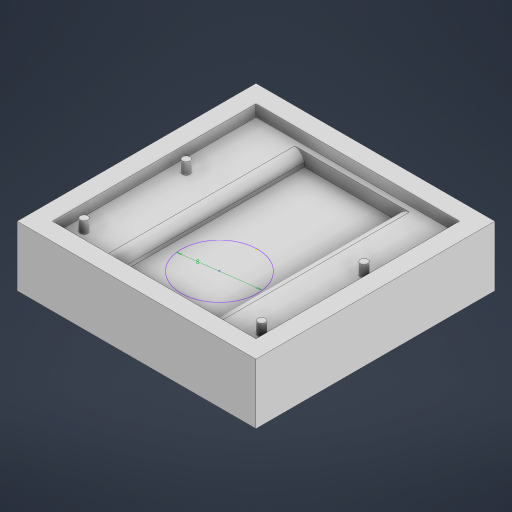
# Autodesk Inventor part: Camera
Saved by Autodesk Inventor 2023.2 (Build 272271030, 271C)
## iProperties
Created: 2025-01-26
Part Number: Camera
Material: Типовые
Document SubType Name: Modeling
Designer: Коноваленко
Density: 1 g/cm^3
Appearance: По умолчанию
Author: Коноваленко
Autodesk Inventor part; units mm, degrees
ref_plane "YZ Plane" through (0, 0, 0) normal (1, 0, 0) x (0, 1, 0)
ref_plane "XZ Plane" through (0, 0, 0) normal (0, 1, 0) x (-1, 0, 0)
ref_plane "XY Plane" through (0, 0, 0) normal (0, 0, 1) x (1, 0, 0)
sketch "Эскиз1" plane through (0, 0, 0) normal (0, 1, 0) x (-1, 0, 0)
  line L0 (12.5, 12.5) -> (-12.5, 12.5)
  line L1 (-12.5, 12.5) -> (-12.5, -12.5)
  line L2 (-12.5, -12.5) -> (12.5, -12.5)
  line L3 (12.5, -12.5) -> (12.5, 12.5)
  line L4 (12.5, 12.5) -> (-12.5, -12.5) construction
  point P0 (0, 0)
  point P1 (0, 0)
  dimension "d0" = 25
  dimension "d1" = 25
  constraints: 10 end point, 2 parallel, 1 coincident, 1 horizontal, 1 midpoint, 1 perpendicular
  measures "d0" distance of L2.end L1.end
  measures "d1" distance of L1.end L0.end
extrude "Выдавливание1" add sketch "Эскиз1" along normal blind 6.3
sketch "Эскиз2" plane through (0, 6.3, 0) normal (0, 1, 0) x (1, 0, 0)
  line L0 (-10.65, -10.65) -> (10.65, -10.65)
  line L1 (10.65, -10.65) -> (10.65, 10.65)
  line L2 (10.65, 10.65) -> (-10.65, 10.65)
  line L3 (-10.65, 10.65) -> (-10.65, -10.65)
  line L4 (-10.65, -10.65) -> (10.65, 10.65) construction
  line L5 (10.65, -10.65) -> (-10.65, 10.65) construction
  line L6 (-12.5, 12.5) -> (-12.5, -12.5) projected
  point P0 (0, 0)
  dimension "d4" = 1.85
  constraints: 12 end point, 2 midpoint, 2 parallel, 2 perpendicular, 1 horizontal
  measures "d4" distance between parallel lines of L3 L6
extrude "Выдавливание2" cut sketch "Эскиз2" against normal blind 1.2
sketch "Эскиз3" plane through (0, 5.1, 0) normal (0, 1, 0) x (1, 0, 0)
  line L0 (5, -9.75) -> (-5, -9.75)
  line L1 (-5, -9.75) -> (-5, 10.05)
  line L2 (-5, 10.05) -> (5, 10.05)
  line L3 (5, 10.05) -> (5, -9.75)
  line L4 (10.65, -10.65) -> (-10.65, -10.65) projected
  line L5 (0, -10.65) -> (0, 6.083) construction
  point P0 (0, 0)
  point P1 (0, -9.75)
  dimension "d7" = 10
  dimension "d8" = 19.8
  dimension "d9" = 0.9
  constraints: 10 end point, 2 midpoint, 2 parallel, 1 horizontal, 1 perpendicular, 1 point on line, 1 vertical
  measures "d7" distance of L1.end L2.end
  measures "d8" distance of L0.end L1.end
  measures "d9" distance between parallel lines of L4 L0
extrude "Выдавливание3" cut sketch "Эскиз3" against normal blind 1.4
fillet "Сопряжение1" radius 1 2 edges at (-5, 5.1, -0.15) (5, 5.1, -0.15)
sketch "Эскиз6" plane through (0, 5.1, 0) normal (0, 1, 0) x (1, 0, 0)
  circle A0 centre (-9.3, 2) radius 0.4
  line L0 (-10.65, -10.65) -> (-10.65, 10.65) projected
  line L1 (-10.65, 10.65) -> (10.65, 10.65) projected
  circle A1 centre (-9.3, -8.7) radius 0.4
  line L2 (10.65, -10.65) -> (-10.65, -10.65) projected
  line L3 (0, -15.7072) -> (0, 17.6357) construction
  circle A2 centre (9.3, 2) radius 0.4
  circle A3 centre (9.3, -8.7) radius 0.4
  point P0 (0, 0)
  dimension "d21" = 0.8
  dimension "d22" = 1.35
  dimension "d23" = 8.65
  dimension "d24" = 0.8
  dimension "d25" = 1.35
  dimension "d26" = 1.55
  constraints: 4 centre point, 2 end point, 2 symmetric about line, 1 vertical, 2 other
  measures "d21" diameter of A0
  measures "d22" distance from line of L0 A0.centre
  measures "d23" distance from line of L1 A0.centre
  measures "d24" diameter of A1
  measures "d25" distance from line of L0 A1.centre
  measures "d26" distance edge to line of A1 L2
extrude "Выдавливание6" add sketch "Эскиз6" along normal blind 1.2
sketch "Эскиз7" plane through (0, 3.7, 0) normal (0, 1, 0) x (1, 0, 0)
  circle A0 centre (0, -3.8434) radius 4
  point P0 (0, 0)
  dimension "d29" = 8
  constraints: 1 centre point
  measures "d29" diameter of A0
